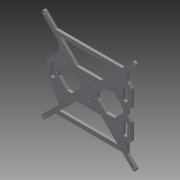
# Autodesk Inventor part: platform_import
Saved by Autodesk Inventor 2015 (Build 190159000, 159)
## iProperties
Created: 2015-04-20
Part Number: platform_import
Material: Generic
Document SubType Name: Modeling
Designer: X
Density: 1 g/cm^3
Appearance: Default
Author: X
Autodesk Inventor part; units mm, degrees
ref_plane "YZ Plane" through (0, 0, 0) normal (1, 0, 0) x (0, 1, 0)
ref_plane "XZ Plane" through (0, 0, 0) normal (0, 1, 0) x (-1, 0, 0)
ref_plane "XY Plane" through (0, 0, 0) normal (0, 0, 1) x (1, 0, 0)
sketch "Sketch1" plane through (0, 0, 0) normal (0, 1, 0) x (-1, 0, 0)
  line L0 (-80.4714, 15.0385) -> (-80.4714, 14.9682)
  line L1 (-100.5417, 4.9682) -> (-120.5417, 24.9682)
  line L2 (-120.5417, 24.9682) -> (-120.5417, 34.9682)
  line L3 (-120.5417, 34.9682) -> (-100.5417, 54.9682)
  line L4 (-100.5417, 54.9682) -> (-90.5417, 54.9682)
  line L5 (-90.5417, 54.9682) -> (-70.5417, 34.9682)
  line L6 (-70.5417, 34.9682) -> (-70.5417, 24.9682)
  line L7 (-70.5417, 24.9682) -> (-90.5417, 4.9682)
  line L8 (-90.5417, 4.9682) -> (-100.5417, 4.9682)
  line L9 (-246.7854, -74.0362) -> (-246.852, -74.5013)
  line L10 (-246.852, -74.5013) -> (-246.7959, -74.9679)
  line L11 (-246.7959, -74.9679) -> (-246.6209, -75.404)
  line L12 (-246.6209, -75.404) -> (-246.339, -75.7799)
  line L13 (-246.339, -75.7799) -> (-245.9695, -76.0701)
  line L14 (-245.9695, -76.0701) -> (-245.5374, -76.2548)
  line L15 (-245.5374, -76.2548) -> (-245.0722, -76.3213)
  line L16 (-245.0722, -76.3213) -> (-244.6057, -76.2652)
  line L17 (-244.6057, -76.2652) -> (-244.1696, -76.0903)
  line L18 (-244.1696, -76.0903) -> (-243.7936, -75.8084)
  line L19 (-243.7936, -75.8084) -> (-243.5034, -75.4388)
  line L20 (-243.5034, -75.4388) -> (-243.3188, -75.0067)
  line L21 (-243.3188, -75.0067) -> (-243.2522, -74.5416)
  line L22 (-243.2522, -74.5416) -> (-243.3083, -74.075)
  line L23 (-243.3083, -74.075) -> (-243.4833, -73.6389)
  line L24 (-243.4833, -73.6389) -> (-243.7652, -73.263)
  line L25 (-243.7652, -73.263) -> (-244.1347, -72.9728)
  line L26 (-244.1347, -72.9728) -> (-244.5668, -72.7881)
  line L27 (-244.5668, -72.7881) -> (-245.032, -72.7216)
  line L28 (-245.032, -72.7216) -> (-245.4985, -72.7777)
  line L29 (-245.4985, -72.7777) -> (-245.9346, -72.9526)
  line L30 (-245.9346, -72.9526) -> (-246.3106, -73.2345)
  line L31 (-246.3106, -73.2345) -> (-246.6008, -73.6041)
  line L32 (-246.6008, -73.6041) -> (-246.7854, -74.0362)
  line L33 (-34.4725, -75.4422) -> (-34.2927, -75.0081)
  line L34 (-34.2927, -75.0081) -> (-34.2314, -74.5422)
  line L35 (-34.2314, -74.5422) -> (-34.2927, -74.0763)
  line L36 (-34.2927, -74.0763) -> (-34.4725, -73.6422)
  line L37 (-34.4725, -73.6422) -> (-34.7586, -73.2694)
  line L38 (-34.7586, -73.2694) -> (-35.1314, -72.9834)
  line L39 (-35.1314, -72.9834) -> (-35.5655, -72.8035)
  line L40 (-35.5655, -72.8035) -> (-36.0314, -72.7422)
  line L41 (-36.0314, -72.7422) -> (-36.4972, -72.8035)
  line L42 (-36.4972, -72.8035) -> (-36.9314, -72.9834)
  line L43 (-36.9314, -72.9834) -> (-37.3041, -73.2694)
  line L44 (-37.3041, -73.2694) -> (-37.5902, -73.6422)
  line L45 (-37.5902, -73.6422) -> (-37.77, -74.0763)
  line L46 (-37.77, -74.0763) -> (-37.8314, -74.5422)
  line L47 (-37.8314, -74.5422) -> (-37.77, -75.0081)
  line L48 (-37.77, -75.0081) -> (-37.5902, -75.4422)
  line L49 (-37.5902, -75.4422) -> (-37.3041, -75.815)
  line L50 (-37.3041, -75.815) -> (-36.9314, -76.1011)
  line L51 (-36.9314, -76.1011) -> (-36.4972, -76.2809)
  line L52 (-36.4972, -76.2809) -> (-36.0314, -76.3422)
  line L53 (-36.0314, -76.3422) -> (-35.5655, -76.2809)
  line L54 (-35.5655, -76.2809) -> (-35.1314, -76.1011)
  line L55 (-35.1314, -76.1011) -> (-34.7586, -75.815)
  line L56 (-34.7586, -75.815) -> (-34.4725, -75.4422)
  line L57 (-35.1314, 132.9197) -> (-34.7586, 133.2057)
  line L58 (-34.7586, 133.2057) -> (-34.4725, 133.5785)
  line L59 (-34.4725, 133.5785) -> (-34.2927, 134.0127)
  line L60 (-34.2927, 134.0127) -> (-34.2314, 134.4785)
  line L61 (-34.2314, 134.4785) -> (-34.2927, 134.9444)
  line L62 (-34.2927, 134.9444) -> (-34.4725, 135.3785)
  line L63 (-34.4725, 135.3785) -> (-34.7586, 135.7513)
  line L64 (-34.7586, 135.7513) -> (-35.1314, 136.0374)
  line L65 (-35.1314, 136.0374) -> (-35.5655, 136.2172)
  line L66 (-35.5655, 136.2172) -> (-36.0314, 136.2785)
  line L67 (-36.0314, 136.2785) -> (-36.4972, 136.2172)
  line L68 (-36.4972, 136.2172) -> (-36.9314, 136.0374)
  line L69 (-36.9314, 136.0374) -> (-37.3041, 135.7513)
  line L70 (-37.3041, 135.7513) -> (-37.5902, 135.3785)
  line L71 (-37.5902, 135.3785) -> (-37.77, 134.9444)
  line L72 (-37.77, 134.9444) -> (-37.8314, 134.4785)
  line L73 (-37.8314, 134.4785) -> (-37.77, 134.0127)
  line L74 (-37.77, 134.0127) -> (-37.5902, 133.5785)
  line L75 (-37.5902, 133.5785) -> (-37.3041, 133.2057)
  line L76 (-37.3041, 133.2057) -> (-36.9314, 132.9197)
  line L77 (-36.9314, 132.9197) -> (-36.4972, 132.7399)
  line L78 (-36.4972, 132.7399) -> (-36.0314, 132.6785)
  line L79 (-36.0314, 132.6785) -> (-35.5655, 132.7399)
  line L80 (-35.5655, 132.7399) -> (-35.1314, 132.9197)
  line L81 (-246.8521, 134.4785) -> (-246.7908, 134.0127)
  line L82 (-246.7908, 134.0127) -> (-246.6109, 133.5785)
  line L83 (-246.6109, 133.5785) -> (-246.3249, 133.2057)
  line L84 (-246.3249, 133.2057) -> (-245.9521, 132.9197)
  line L85 (-245.9521, 132.9197) -> (-245.518, 132.7399)
  line L86 (-245.518, 132.7399) -> (-245.0521, 132.6785)
  line L87 (-245.0521, 132.6785) -> (-244.5862, 132.7399)
  line L88 (-244.5862, 132.7399) -> (-244.1521, 132.9197)
  line L89 (-244.1521, 132.9197) -> (-243.7793, 133.2057)
  line L90 (-243.7793, 133.2057) -> (-243.4933, 133.5785)
  line L91 (-243.4933, 133.5785) -> (-243.3134, 134.0127)
  line L92 (-243.3134, 134.0127) -> (-243.2521, 134.4785)
  line L93 (-243.2521, 134.4785) -> (-243.3134, 134.9444)
  line L94 (-243.3134, 134.9444) -> (-243.4933, 135.3785)
  line L95 (-243.4933, 135.3785) -> (-243.7793, 135.7513)
  line L96 (-243.7793, 135.7513) -> (-244.1521, 136.0374)
  line L97 (-244.1521, 136.0374) -> (-244.5862, 136.2172)
  line L98 (-244.5862, 136.2172) -> (-245.0521, 136.2785)
  line L99 (-245.0521, 136.2785) -> (-245.4714, 136.2181)
  line L100 (-245.4714, 136.2181) -> (-245.518, 136.2172)
  line L101 (-245.518, 136.2172) -> (-245.9521, 136.0374)
  line L102 (-245.9521, 136.0374) -> (-246.3249, 135.7513)
  line L103 (-246.3249, 135.7513) -> (-246.6109, 135.3785)
  line L104 (-246.6109, 135.3785) -> (-246.7908, 134.9444)
  line L105 (-246.7908, 134.9444) -> (-246.8521, 134.4785)
  line L106 (-142.0634, 49.0541) -> (-141.7773, 48.6814)
  line L107 (-141.7773, 48.6814) -> (-141.4045, 48.3954)
  line L108 (-141.4045, 48.3954) -> (-140.9703, 48.2156)
  line L109 (-140.9703, 48.2156) -> (-140.5045, 48.1544)
  line L110 (-140.5045, 48.1544) -> (-140.0386, 48.2158)
  line L111 (-140.0386, 48.2158) -> (-139.6045, 48.3956)
  line L112 (-139.6045, 48.3956) -> (-139.2317, 48.6817)
  line L113 (-139.2317, 48.6817) -> (-138.9457, 49.0546)
  line L114 (-138.9457, 49.0546) -> (-138.766, 49.4887)
  line L115 (-138.766, 49.4887) -> (-138.7047, 49.9546)
  line L116 (-138.7047, 49.9546) -> (-138.7661, 50.4205)
  line L117 (-138.7661, 50.4205) -> (-138.946, 50.8546)
  line L118 (-138.946, 50.8546) -> (-139.2321, 51.2273)
  line L119 (-139.2321, 51.2273) -> (-139.6049, 51.5133)
  line L120 (-139.6049, 51.5133) -> (-140.0391, 51.6931)
  line L121 (-140.0391, 51.6931) -> (-140.505, 51.7544)
  line L122 (-140.505, 51.7544) -> (-140.9708, 51.693)
  line L123 (-140.9708, 51.693) -> (-141.4049, 51.5131)
  line L124 (-141.4049, 51.5131) -> (-141.7777, 51.227)
  line L125 (-141.7777, 51.227) -> (-142.0637, 50.8541)
  line L126 (-142.0637, 50.8541) -> (-142.2434, 50.42)
  line L127 (-142.2434, 50.42) -> (-142.3047, 49.9541)
  line L128 (-142.3047, 49.9541) -> (-142.2433, 49.4882)
  line L129 (-142.2433, 49.4882) -> (-142.0634, 49.0541)
  line L130 (-45.93, 31.417) -> (-46.2917, 31.2672)
  line L131 (-46.2917, 31.2672) -> (-46.6024, 31.0288)
  line L132 (-46.6024, 31.0288) -> (-46.8408, 30.7182)
  line L133 (-46.8408, 30.7182) -> (-46.9906, 30.3564)
  line L134 (-46.9906, 30.3564) -> (-47.0417, 29.9682)
  line L135 (-47.0417, 29.9682) -> (-46.9906, 29.5799)
  line L136 (-46.9906, 29.5799) -> (-46.8408, 29.2182)
  line L137 (-46.8408, 29.2182) -> (-46.6024, 28.9075)
  line L138 (-46.6024, 28.9075) -> (-46.2917, 28.6691)
  line L139 (-46.2917, 28.6691) -> (-45.93, 28.5193)
  line L140 (-45.93, 28.5193) -> (-45.5417, 28.4682)
  line L141 (-45.5417, 28.4682) -> (-45.1535, 28.5193)
  line L142 (-45.1535, 28.5193) -> (-44.7917, 28.6691)
  line L143 (-44.7917, 28.6691) -> (-44.4811, 28.9075)
  line L144 (-44.4811, 28.9075) -> (-44.2427, 29.2182)
  line L145 (-44.2427, 29.2182) -> (-44.0928, 29.5799)
  line L146 (-44.0928, 29.5799) -> (-44.0417, 29.9682)
  line L147 (-44.0417, 29.9682) -> (-44.0928, 30.3564)
  line L148 (-44.0928, 30.3564) -> (-44.2427, 30.7182)
  line L149 (-44.2427, 30.7182) -> (-44.4811, 31.0288)
  line L150 (-44.4811, 31.0288) -> (-44.7917, 31.2672)
  line L151 (-44.7917, 31.2672) -> (-45.1535, 31.417)
  line L152 (-45.1535, 31.417) -> (-45.5417, 31.4682)
  line L153 (-45.5417, 31.4682) -> (-45.93, 31.417)
  line L154 (-180.5417, 54.9682) -> (-160.5417, 34.9682)
  line L155 (-160.5417, 34.9682) -> (-160.5417, 24.9682)
  line L156 (-160.5417, 24.9682) -> (-180.5417, 4.9682)
  line L157 (-180.5417, 4.9682) -> (-200.5417, 4.9682)
  line L158 (-200.5417, 4.9682) -> (-220.5417, 24.9682)
  line L159 (-220.5417, 24.9682) -> (-220.5417, 34.9682)
  line L160 (-220.5417, 34.9682) -> (-200.5417, 54.9682)
  line L161 (-200.5417, 54.9682) -> (-180.4714, 54.9682)
  line L162 (-234.0417, 64.9682) -> (-234.0928, 65.3564)
  line L163 (-234.0928, 65.3564) -> (-234.2427, 65.7182)
  line L164 (-234.2427, 65.7182) -> (-234.4811, 66.0288)
  line L165 (-234.4811, 66.0288) -> (-234.7917, 66.2672)
  line L166 (-234.7917, 66.2672) -> (-235.1535, 66.417)
  line L167 (-235.1535, 66.417) -> (-235.5417, 66.4682)
  line L168 (-235.5417, 66.4682) -> (-235.9299, 66.417)
  line L169 (-235.9299, 66.417) -> (-236.2917, 66.2672)
  line L170 (-236.2917, 66.2672) -> (-236.6024, 66.0288)
  line L171 (-236.6024, 66.0288) -> (-236.8408, 65.7182)
  line L172 (-236.8408, 65.7182) -> (-236.9906, 65.3564)
  line L173 (-236.9906, 65.3564) -> (-237.0417, 64.9682)
  line L174 (-237.0417, 64.9682) -> (-236.9906, 64.5799)
  line L175 (-236.9906, 64.5799) -> (-236.8408, 64.2182)
  line L176 (-236.8408, 64.2182) -> (-236.6024, 63.9075)
  line L177 (-236.6024, 63.9075) -> (-236.2917, 63.6691)
  line L178 (-236.2917, 63.6691) -> (-235.9299, 63.5193)
  line L179 (-235.9299, 63.5193) -> (-235.5417, 63.4682)
  line L180 (-235.5417, 63.4682) -> (-235.1535, 63.5193)
  line L181 (-235.1535, 63.5193) -> (-234.7917, 63.6691)
  line L182 (-234.7917, 63.6691) -> (-234.4811, 63.9075)
  line L183 (-234.4811, 63.9075) -> (-234.2427, 64.2182)
  line L184 (-234.2427, 64.2182) -> (-234.0928, 64.5799)
  line L185 (-234.0928, 64.5799) -> (-234.0417, 64.9682)
  line L186 (-58.5417, 14.3669) -> (-58.0725, 14.1355)
  line L187 (-58.0725, 14.1355) -> (-57.577, 13.9673)
  line L188 (-57.577, 13.9673) -> (-57.0638, 13.8653)
  line L189 (-57.0638, 13.8653) -> (-56.5417, 13.831)
  line L190 (-56.5417, 13.831) -> (-54.5417, 13.831)
  line L191 (-54.5417, 13.831) -> (-54.0196, 13.8653)
  line L192 (-54.0196, 13.8653) -> (-53.5065, 13.9673)
  line L193 (-53.5065, 13.9673) -> (-53.011, 14.1355)
  line L194 (-53.011, 14.1355) -> (-52.5417, 14.3669)
  line L195 (-52.5417, 14.3669) -> (-52.1067, 14.6576)
  line L196 (-52.1067, 14.6576) -> (-51.7133, 15.0026)
  line L197 (-51.7133, 15.0026) -> (-51.3683, 15.396)
  line L198 (-51.3683, 15.396) -> (-51.0776, 15.831)
  line L199 (-51.0776, 15.831) -> (-50.8462, 16.3003)
  line L200 (-50.8462, 16.3003) -> (-50.678, 16.7958)
  line L201 (-50.678, 16.7958) -> (-50.576, 17.3089)
  line L202 (-50.576, 17.3089) -> (-50.5417, 17.831)
  line L203 (-50.5417, 17.831) -> (-50.5417, 40.831)
  line L204 (-50.5417, 40.831) -> (-50.576, 41.3531)
  line L205 (-50.576, 41.3531) -> (-50.678, 41.8663)
  line L206 (-50.678, 41.8663) -> (-50.8462, 42.3618)
  line L207 (-50.8462, 42.3618) -> (-51.0776, 42.831)
  line L208 (-51.0776, 42.831) -> (-51.3683, 43.2661)
  line L209 (-51.3683, 43.2661) -> (-51.7133, 43.6595)
  line L210 (-51.7133, 43.6595) -> (-52.1067, 44.0044)
  line L211 (-52.1067, 44.0044) -> (-52.5417, 44.2951)
  line L212 (-52.5417, 44.2951) -> (-53.011, 44.5266)
  line L213 (-53.011, 44.5266) -> (-53.5065, 44.6947)
  line L214 (-53.5065, 44.6947) -> (-54.0196, 44.7968)
  line L215 (-54.0196, 44.7968) -> (-54.5417, 44.831)
  line L216 (-54.5417, 44.831) -> (-56.5417, 44.831)
  line L217 (-56.5417, 44.831) -> (-57.0638, 44.7968)
  line L218 (-57.0638, 44.7968) -> (-57.577, 44.6947)
  line L219 (-57.577, 44.6947) -> (-58.0725, 44.5266)
  line L220 (-58.0725, 44.5266) -> (-58.5417, 44.2951)
  line L221 (-58.5417, 44.2951) -> (-58.9768, 44.0044)
  line L222 (-58.9768, 44.0044) -> (-59.3702, 43.6595)
  line L223 (-59.3702, 43.6595) -> (-59.7151, 43.2661)
  line L224 (-59.7151, 43.2661) -> (-60.0058, 42.831)
  line L225 (-60.0058, 42.831) -> (-60.2373, 42.3618)
  line L226 (-60.2373, 42.3618) -> (-60.4054, 41.8663)
  line L227 (-60.4054, 41.8663) -> (-60.5075, 41.3531)
  line L228 (-60.5075, 41.3531) -> (-60.5417, 40.831)
  line L229 (-60.5417, 40.831) -> (-60.5417, 17.831)
  line L230 (-60.5417, 17.831) -> (-60.5075, 17.3089)
  line L231 (-60.5075, 17.3089) -> (-60.4054, 16.7958)
  line L232 (-60.4054, 16.7958) -> (-60.2373, 16.3003)
  line L233 (-60.2373, 16.3003) -> (-60.0058, 15.831)
  line L234 (-60.0058, 15.831) -> (-59.7151, 15.396)
  line L235 (-59.7151, 15.396) -> (-59.3702, 15.0026)
  line L236 (-59.3702, 15.0026) -> (-58.9768, 14.6576)
  line L237 (-58.9768, 14.6576) -> (-58.5417, 14.3669)
  line L238 (-66.8408, 30.7182) -> (-66.9906, 30.3564)
  line L239 (-66.9906, 30.3564) -> (-67.0417, 29.9682)
  line L240 (-67.0417, 29.9682) -> (-66.9906, 29.5799)
  line L241 (-66.9906, 29.5799) -> (-66.8408, 29.2182)
  line L242 (-66.8408, 29.2182) -> (-66.6024, 28.9075)
  line L243 (-66.6024, 28.9075) -> (-66.2917, 28.6691)
  line L244 (-66.2917, 28.6691) -> (-65.93, 28.5193)
  line L245 (-65.93, 28.5193) -> (-65.5417, 28.4682)
  line L246 (-65.5417, 28.4682) -> (-65.1535, 28.5193)
  line L247 (-65.1535, 28.5193) -> (-64.7917, 28.6691)
  line L248 (-64.7917, 28.6691) -> (-64.4811, 28.9075)
  line L249 (-64.4811, 28.9075) -> (-64.2427, 29.2182)
  line L250 (-64.2427, 29.2182) -> (-64.0928, 29.5799)
  line L251 (-64.0928, 29.5799) -> (-64.0417, 29.9682)
  line L252 (-64.0417, 29.9682) -> (-64.0928, 30.3564)
  line L253 (-64.0928, 30.3564) -> (-64.2427, 30.7182)
  line L254 (-64.2427, 30.7182) -> (-64.4811, 31.0288)
  line L255 (-64.4811, 31.0288) -> (-64.7917, 31.2672)
  line L256 (-64.7917, 31.2672) -> (-65.1535, 31.417)
  line L257 (-65.1535, 31.417) -> (-65.5417, 31.4682)
  line L258 (-65.5417, 31.4682) -> (-65.93, 31.417)
  line L259 (-65.93, 31.417) -> (-66.2917, 31.2672)
  line L260 (-66.2917, 31.2672) -> (-66.6024, 31.0288)
  line L261 (-66.6024, 31.0288) -> (-66.8408, 30.7182)
  line L262 (-72.4714, 104.9682) -> (-112.4714, 64.9682)
  line L263 (-112.4714, 64.9682) -> (-168.5417, 64.9682)
  line L264 (-168.5417, 64.9682) -> (-208.5417, 104.9682)
  line L265 (-208.5417, 104.9682) -> (-72.4714, 104.9682)
  line L266 (-215.1535, -3.583) -> (-215.5417, -3.5318)
  line L267 (-215.5417, -3.5318) -> (-215.9299, -3.583)
  line L268 (-215.9299, -3.583) -> (-216.2917, -3.7328)
  line L269 (-216.2917, -3.7328) -> (-216.6024, -3.9712)
  line L270 (-216.6024, -3.9712) -> (-216.8408, -4.2818)
  line L271 (-216.8408, -4.2818) -> (-216.9906, -4.6436)
  line L272 (-216.9906, -4.6436) -> (-217.0417, -5.0318)
  line L273 (-217.0417, -5.0318) -> (-216.9906, -5.4201)
  line L274 (-216.9906, -5.4201) -> (-216.8408, -5.7818)
  line L275 (-216.8408, -5.7818) -> (-216.6024, -6.0925)
  line L276 (-216.6024, -6.0925) -> (-216.2917, -6.3309)
  line L277 (-216.2917, -6.3309) -> (-215.9299, -6.4807)
  line L278 (-215.9299, -6.4807) -> (-215.5417, -6.5318)
  line L279 (-215.5417, -6.5318) -> (-215.1535, -6.4807)
  line L280 (-215.1535, -6.4807) -> (-214.7917, -6.3309)
  line L281 (-214.7917, -6.3309) -> (-214.4811, -6.0925)
  line L282 (-214.4811, -6.0925) -> (-214.2427, -5.7818)
  line L283 (-214.2427, -5.7818) -> (-214.0928, -5.4201)
  line L284 (-214.0928, -5.4201) -> (-214.0417, -5.0318)
  line L285 (-214.0417, -5.0318) -> (-214.0928, -4.6436)
  line L286 (-214.0928, -4.6436) -> (-214.2427, -4.2818)
  line L287 (-214.2427, -4.2818) -> (-214.4811, -3.9712)
  line L288 (-214.4811, -3.9712) -> (-214.7917, -3.7328)
  line L289 (-214.7917, -3.7328) -> (-215.1535, -3.583)
  line L290 (-230.2372, 8.4989) -> (-230.4054, 8.0034)
  line L291 (-230.4054, 8.0034) -> (-230.5075, 7.4903)
  line L292 (-230.5075, 7.4903) -> (-230.5417, 6.9682)
  line L293 (-230.5417, 6.9682) -> (-230.5417, -16.0318)
  line L294 (-230.5417, -16.0318) -> (-230.5075, -16.5539)
  line L295 (-230.5075, -16.5539) -> (-230.4054, -17.0671)
  line L296 (-230.4054, -17.0671) -> (-230.2372, -17.5626)
  line L297 (-230.2372, -17.5626) -> (-230.0058, -18.0318)
  line L298 (-230.0058, -18.0318) -> (-229.7151, -18.4669)
  line L299 (-229.7151, -18.4669) -> (-229.3701, -18.8603)
  line L300 (-229.3701, -18.8603) -> (-228.9768, -19.2053)
  line L301 (-228.9768, -19.2053) -> (-228.5417, -19.4959)
  line L302 (-228.5417, -19.4959) -> (-228.0725, -19.7274)
  line L303 (-228.0725, -19.7274) -> (-227.577, -19.8955)
  line L304 (-227.577, -19.8955) -> (-227.0638, -19.9976)
  line L305 (-227.0638, -19.9976) -> (-226.5417, -20.0318)
  line L306 (-226.5417, -20.0318) -> (-224.5417, -20.0318)
  line L307 (-224.5417, -20.0318) -> (-224.0196, -19.9976)
  line L308 (-224.0196, -19.9976) -> (-223.5064, -19.8955)
  line L309 (-223.5064, -19.8955) -> (-223.011, -19.7274)
  line L310 (-223.011, -19.7274) -> (-222.5417, -19.4959)
  line L311 (-222.5417, -19.4959) -> (-222.1067, -19.2053)
  line L312 (-222.1067, -19.2053) -> (-221.7133, -18.8603)
  line L313 (-221.7133, -18.8603) -> (-221.3683, -18.4669)
  line L314 (-221.3683, -18.4669) -> (-221.0776, -18.0318)
  line L315 (-221.0776, -18.0318) -> (-220.8462, -17.5626)
  line L316 (-220.8462, -17.5626) -> (-220.678, -17.0671)
  line L317 (-220.678, -17.0671) -> (-220.5759, -16.5539)
  line L318 (-220.5759, -16.5539) -> (-220.5417, -16.0318)
  line L319 (-220.5417, -16.0318) -> (-220.5417, 6.9682)
  line L320 (-220.5417, 6.9682) -> (-220.5759, 7.4903)
  line L321 (-220.5759, 7.4903) -> (-220.678, 8.0034)
  line L322 (-220.678, 8.0034) -> (-220.8462, 8.4989)
  line L323 (-220.8462, 8.4989) -> (-221.0776, 8.9682)
  line L324 (-221.0776, 8.9682) -> (-221.3683, 9.4032)
  line L325 (-221.3683, 9.4032) -> (-221.7133, 9.7966)
  line L326 (-221.7133, 9.7966) -> (-222.1067, 10.1416)
  line L327 (-222.1067, 10.1416) -> (-222.5417, 10.4323)
  line L328 (-222.5417, 10.4323) -> (-223.011, 10.6637)
  line L329 (-223.011, 10.6637) -> (-223.5064, 10.8319)
  line L330 (-223.5064, 10.8319) -> (-224.0196, 10.9339)
  line L331 (-224.0196, 10.9339) -> (-224.5417, 10.9682)
  line L332 (-224.5417, 10.9682) -> (-226.5417, 10.9682)
  line L333 (-226.5417, 10.9682) -> (-227.0638, 10.9339)
  line L334 (-227.0638, 10.9339) -> (-227.577, 10.8319)
  line L335 (-227.577, 10.8319) -> (-228.0725, 10.6637)
  line L336 (-228.0725, 10.6637) -> (-228.5417, 10.4323)
  line L337 (-228.5417, 10.4323) -> (-228.9768, 10.1416)
  line L338 (-228.9768, 10.1416) -> (-229.3701, 9.7966)
  line L339 (-229.3701, 9.7966) -> (-229.7151, 9.4032)
  line L340 (-229.7151, 9.4032) -> (-230.0058, 8.9682)
  line L341 (-230.0058, 8.9682) -> (-230.2372, 8.4989)
  line L342 (-214.0928, 65.3564) -> (-214.2427, 65.7182)
  line L343 (-214.2427, 65.7182) -> (-214.4811, 66.0288)
  line L344 (-214.4811, 66.0288) -> (-214.7917, 66.2672)
  line L345 (-214.7917, 66.2672) -> (-215.1535, 66.417)
  line L346 (-215.1535, 66.417) -> (-215.5417, 66.4682)
  line L347 (-215.5417, 66.4682) -> (-215.9299, 66.417)
  line L348 (-215.9299, 66.417) -> (-216.2917, 66.2672)
  line L349 (-216.2917, 66.2672) -> (-216.6024, 66.0288)
  line L350 (-216.6024, 66.0288) -> (-216.8408, 65.7182)
  line L351 (-216.8408, 65.7182) -> (-216.9906, 65.3564)
  line L352 (-216.9906, 65.3564) -> (-217.0417, 64.9682)
  line L353 (-217.0417, 64.9682) -> (-216.9906, 64.5799)
  line L354 (-216.9906, 64.5799) -> (-216.8408, 64.2182)
  line L355 (-216.8408, 64.2182) -> (-216.6024, 63.9075)
  line L356 (-216.6024, 63.9075) -> (-216.2917, 63.6691)
  line L357 (-216.2917, 63.6691) -> (-215.9299, 63.5193)
  line L358 (-215.9299, 63.5193) -> (-215.5417, 63.4682)
  line L359 (-215.5417, 63.4682) -> (-215.1535, 63.5193)
  line L360 (-215.1535, 63.5193) -> (-214.7917, 63.6691)
  line L361 (-214.7917, 63.6691) -> (-214.4811, 63.9075)
  line L362 (-214.4811, 63.9075) -> (-214.2427, 64.2182)
  line L363 (-214.2427, 64.2182) -> (-214.0928, 64.5799)
  line L364 (-214.0928, 64.5799) -> (-214.0417, 64.9682)
  line L365 (-214.0417, 64.9682) -> (-214.0928, 65.3564)
  line L366 (-228.5417, 80.4393) -> (-228.0725, 80.6707)
  line L367 (-228.0725, 80.6707) -> (-227.577, 80.8389)
  line L368 (-227.577, 80.8389) -> (-227.0638, 80.941)
  line L369 (-227.0638, 80.941) -> (-226.5417, 80.9752)
  line L370 (-226.5417, 80.9752) -> (-224.5417, 80.9752)
  line L371 (-224.5417, 80.9752) -> (-224.0196, 80.941)
  line L372 (-224.0196, 80.941) -> (-223.5064, 80.8389)
  line L373 (-223.5064, 80.8389) -> (-223.011, 80.6707)
  line L374 (-223.011, 80.6707) -> (-222.5417, 80.4393)
  line L375 (-222.5417, 80.4393) -> (-222.1067, 80.1486)
  line L376 (-222.1067, 80.1486) -> (-221.7133, 79.8036)
  line L377 (-221.7133, 79.8036) -> (-221.3683, 79.4102)
  line L378 (-221.3683, 79.4102) -> (-221.0776, 78.9752)
  line L379 (-221.0776, 78.9752) -> (-220.8462, 78.5059)
  line L380 (-220.8462, 78.5059) -> (-220.678, 78.0105)
  line L381 (-220.678, 78.0105) -> (-220.5759, 77.4973)
  line L382 (-220.5759, 77.4973) -> (-220.5417, 76.9752)
  line L383 (-220.5417, 76.9752) -> (-220.5417, 53.9752)
  line L384 (-220.5417, 53.9752) -> (-220.5759, 53.4531)
  line L385 (-220.5759, 53.4531) -> (-220.678, 52.9399)
  line L386 (-220.678, 52.9399) -> (-220.8462, 52.4445)
  line L387 (-220.8462, 52.4445) -> (-221.0776, 51.9752)
  line L388 (-221.0776, 51.9752) -> (-221.3683, 51.5401)
  line L389 (-221.3683, 51.5401) -> (-221.7133, 51.1468)
  line L390 (-221.7133, 51.1468) -> (-222.1067, 50.8018)
  line L391 (-222.1067, 50.8018) -> (-222.5417, 50.5111)
  line L392 (-222.5417, 50.5111) -> (-223.011, 50.2797)
  line L393 (-223.011, 50.2797) -> (-223.5064, 50.1115)
  line L394 (-223.5064, 50.1115) -> (-224.0196, 50.0094)
  line L395 (-224.0196, 50.0094) -> (-224.5417, 49.9752)
  line L396 (-224.5417, 49.9752) -> (-226.5417, 49.9752)
  line L397 (-226.5417, 49.9752) -> (-227.0638, 50.0094)
  line L398 (-227.0638, 50.0094) -> (-227.577, 50.1115)
  line L399 (-227.577, 50.1115) -> (-228.0725, 50.2797)
  line L400 (-228.0725, 50.2797) -> (-228.5417, 50.5111)
  line L401 (-228.5417, 50.5111) -> (-228.9768, 50.8018)
  line L402 (-228.9768, 50.8018) -> (-229.3701, 51.1468)
  line L403 (-229.3701, 51.1468) -> (-229.7151, 51.5401)
  line L404 (-229.7151, 51.5401) -> (-230.0058, 51.9752)
  line L405 (-230.0058, 51.9752) -> (-230.2372, 52.4445)
  line L406 (-230.2372, 52.4445) -> (-230.4054, 52.9399)
  line L407 (-230.4054, 52.9399) -> (-230.5075, 53.4531)
  line L408 (-230.5075, 53.4531) -> (-230.5417, 53.9752)
  line L409 (-230.5417, 53.9752) -> (-230.5417, 76.9752)
  line L410 (-230.5417, 76.9752) -> (-230.5075, 77.4973)
  line L411 (-230.5075, 77.4973) -> (-230.4054, 78.0105)
  line L412 (-230.4054, 78.0105) -> (-230.2372, 78.5059)
  line L413 (-230.2372, 78.5059) -> (-230.0058, 78.9752)
  line L414 (-230.0058, 78.9752) -> (-229.7151, 79.4102)
  line L415 (-229.7151, 79.4102) -> (-229.3701, 79.8036)
  line L416 (-229.3701, 79.8036) -> (-228.9768, 80.1486)
  line L417 (-228.9768, 80.1486) -> (-228.5417, 80.4393)
  line L418 (-37.5417, 139.9681) -> (-62.5417, 114.9682)
  line L419 (-62.5417, 114.9682) -> (-218.5417, 114.9682)
  line L420 (-218.5417, 114.9682) -> (-243.5417, 139.9681)
  line L421 (-243.5417, 139.9681) -> (-247.5417, 139.9681)
  line L422 (-247.5417, 139.9681) -> (-250.5417, 136.9681)
  line L423 (-250.5417, 136.9681) -> (-250.5417, 132.9681)
  line L424 (-250.5417, 132.9681) -> (-230.5417, 112.9682)
  line L425 (-230.5417, 112.9682) -> (-230.5417, 92.9682)
  line L426 (-230.5417, 92.9682) -> (-240.5417, 82.9682)
  line L427 (-240.5417, 82.9682) -> (-240.5417, 44.9682)
  line L428 (-240.5417, 44.9682) -> (-230.5417, 34.9682)
  line L429 (-230.5417, 34.9682) -> (-230.5417, 24.9682)
  line L430 (-230.5417, 24.9682) -> (-240.5417, 14.9682)
  line L431 (-240.5417, 14.9682) -> (-240.5417, -23.0318)
  line L432 (-240.5417, -23.0318) -> (-230.5417, -33.0318)
  line L433 (-230.5417, -33.0318) -> (-230.5417, -53.0318)
  line L434 (-230.5417, -53.0318) -> (-250.5417, -73.0318)
  line L435 (-250.5417, -73.0318) -> (-250.5417, -77.0318)
  line L436 (-250.5417, -77.0318) -> (-247.5417, -80.0318)
  line L437 (-247.5417, -80.0318) -> (-243.5417, -80.0318)
  line L438 (-243.5417, -80.0318) -> (-218.5417, -55.0318)
  line L439 (-218.5417, -55.0318) -> (-62.5417, -55.0318)
  line L440 (-62.5417, -55.0318) -> (-37.5417, -80.0318)
  line L441 (-37.5417, -80.0318) -> (-33.5417, -80.0318)
  line L442 (-33.5417, -80.0318) -> (-30.5417, -77.0318)
  line L443 (-30.5417, -77.0318) -> (-30.5417, -73.0318)
  line L444 (-30.5417, -73.0318) -> (-50.5417, -53.0318)
  line L445 (-50.5417, -53.0318) -> (-70.5417, -33.0318)
  line L446 (-70.5417, -33.0318) -> (-50.5417, 6.9682)
  line L447 (-50.5417, 6.9682) -> (-40.5417, 16.9682)
  line L448 (-40.5417, 16.9682) -> (-40.5417, 42.9682)
  line L449 (-40.5417, 42.9682) -> (-50.5417, 52.9682)
  line L450 (-50.5417, 52.9682) -> (-70.5417, 72.9682)
  line L451 (-70.5417, 72.9682) -> (-70.5417, 92.9682)
  line L452 (-70.5417, 92.9682) -> (-30.5417, 132.9681)
  line L453 (-30.5417, 132.9681) -> (-30.5417, 136.9681)
  line L454 (-30.5417, 136.9681) -> (-33.5417, 139.9681)
  line L455 (-33.5417, 139.9681) -> (-37.5417, 139.9681)
  line L456 (-236.8408, -5.7818) -> (-236.6024, -6.0925)
  line L457 (-236.6024, -6.0925) -> (-236.2917, -6.3309)
  line L458 (-236.2917, -6.3309) -> (-235.9299, -6.4807)
  line L459 (-235.9299, -6.4807) -> (-235.5417, -6.5318)
  line L460 (-235.5417, -6.5318) -> (-235.1535, -6.4807)
  line L461 (-235.1535, -6.4807) -> (-234.7917, -6.3309)
  line L462 (-234.7917, -6.3309) -> (-234.4811, -6.0925)
  line L463 (-234.4811, -6.0925) -> (-234.2427, -5.7818)
  line L464 (-234.2427, -5.7818) -> (-234.0928, -5.4201)
  line L465 (-234.0928, -5.4201) -> (-234.0417, -5.0318)
  line L466 (-234.0417, -5.0318) -> (-234.0928, -4.6436)
  line L467 (-234.0928, -4.6436) -> (-234.2427, -4.2818)
  line L468 (-234.2427, -4.2818) -> (-234.4811, -3.9712)
  line L469 (-234.4811, -3.9712) -> (-234.7917, -3.7328)
  line L470 (-234.7917, -3.7328) -> (-235.1535, -3.583)
  line L471 (-235.1535, -3.583) -> (-235.5417, -3.5318)
  line L472 (-235.5417, -3.5318) -> (-235.9299, -3.583)
  line L473 (-235.9299, -3.583) -> (-236.2917, -3.7328)
  line L474 (-236.2917, -3.7328) -> (-236.6024, -3.9712)
  line L475 (-236.6024, -3.9712) -> (-236.8408, -4.2818)
  line L476 (-236.8408, -4.2818) -> (-236.9906, -4.6436)
  line L477 (-236.9906, -4.6436) -> (-237.0417, -5.0318)
  line L478 (-237.0417, -5.0318) -> (-236.9906, -5.4201)
  line L479 (-236.9906, -5.4201) -> (-236.8408, -5.7818)
  line L480 (-140.9708, 10.7132) -> (-141.4049, 10.5333)
  line L481 (-141.4049, 10.5333) -> (-141.7777, 10.2472)
  line L482 (-141.7777, 10.2472) -> (-142.0637, 9.8743)
  line L483 (-142.0637, 9.8743) -> (-142.2434, 9.4402)
  line L484 (-142.2434, 9.4402) -> (-142.3047, 8.9743)
  line L485 (-142.3047, 8.9743) -> (-142.2433, 8.5084)
  line L486 (-142.2433, 8.5084) -> (-142.0634, 8.0743)
  line L487 (-142.0634, 8.0743) -> (-141.7773, 7.7016)
  line L488 (-141.7773, 7.7016) -> (-141.4045, 7.4156)
  line L489 (-141.4045, 7.4156) -> (-140.9703, 7.2358)
  line L490 (-140.9703, 7.2358) -> (-140.5045, 7.1746)
  line L491 (-140.5045, 7.1746) -> (-140.0386, 7.236)
  line L492 (-140.0386, 7.236) -> (-139.6045, 7.4158)
  line L493 (-139.6045, 7.4158) -> (-139.2317, 7.702)
  line L494 (-139.2317, 7.702) -> (-138.9457, 8.0748)
  line L495 (-138.9457, 8.0748) -> (-138.766, 8.5089)
  line L496 (-138.766, 8.5089) -> (-138.7047, 8.9748)
  line L497 (-138.7047, 8.9748) -> (-138.7661, 9.4407)
  line L498 (-138.7661, 9.4407) -> (-138.946, 9.8748)
  line L499 (-138.946, 9.8748) -> (-139.2321, 10.2475)
  line L500 (-139.2321, 10.2475) -> (-139.6049, 10.5335)
  line L501 (-139.6049, 10.5335) -> (-140.0391, 10.7133)
  line L502 (-140.0391, 10.7133) -> (-140.505, 10.7746)
  line L503 (-140.505, 10.7746) -> (-140.9708, 10.7132)
  line L504 (-80.4714, 44.9682) -> (-80.4714, 44.8978)
  line L505 (-112.5417, -5.0318) -> (-72.5417, -45.0318)
  line L506 (-168.5417, -5.0318) -> (-112.4714, -5.0318)
  line L507 (-112.4714, -5.0318) -> (-72.4714, -45.0318)
  line L508 (-72.4714, -45.0318) -> (-208.5417, -45.0318)
  line L509 (-208.5417, -45.0318) -> (-168.5417, -5.0318)
  constraints: 1020 end point, 5 point on line
extrude "Extrusion1" add sketch "Sketch1" along normal blind 6
body "Solid1"
